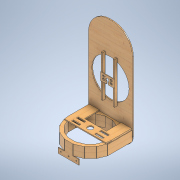
# Autodesk Inventor part: Aufbau
Saved by Autodesk Inventor 2020.3 (Build 243373010, 373A)
## iProperties
Created: 2020-02-10
Part Number: Aufbau
Material: Generisch
Document SubType Name: Modeling
Designer: Stefan
Density: 1 g/cm^3
Appearance: Vorgabe
Mass: 38281.1 g
Surface Area: 55122.2 cm^2
Volume: 38281.1 cm^3
Author: Stefan
Autodesk Inventor part; units mm, degrees
ref_plane "YZ Plane" through (0, 0, 0) normal (1, 0, 0) x (0, 1, 0)
ref_plane "XZ Plane" through (0, 0, 0) normal (0, 1, 0) x (-1, 0, 0)
ref_plane "XY Plane" through (0, 0, 0) normal (0, 0, 1) x (1, 0, 0)
sketch "Skizze1" plane through (0, 0, 0) normal (0, 0, 1) x (-1, 0, 0)
  line L0 (225, 975) -> (-225, 975)
  line L1 (-425, 775) -> (-425, -575)
  line L2 (-25, -975) -> (25, -975)
  line L3 (425, -575) -> (425, 775)
  arc A0 (425, 775) -> (225, 975) centre (225, 775) ccw
  arc A1 (-225, 975) -> (-425, 775) centre (-225, 775) ccw
  arc A2 (-425, -575) -> (-25, -975) centre (-25, -575) ccw
  arc A3 (25, -975) -> (425, -575) centre (25, -575) ccw
  circle A4 centre (0, 0) radius 360
  point P0 (425, 975)
  point P1 (-425, 975)
  point P2 (425, -975)
  dimension "d0" = 850
  dimension "d1" = 1950
  dimension "d2" = 975
  dimension "d3" = 425
  dimension "d4" = 200
  dimension "d5" = 200
  dimension "d6" = 400
  dimension "d7" = 400
  dimension "d8" = 720
  constraints: 8 end point, 8 point on circle, 8 tangent, 6 point on line, 5 centre point, 2 parallel, 1 coincident, 1 horizontal, 1 perpendicular
  measures "d0" distance of point (425, 975) point (-425, 975)
  measures "d1" distance of point (425, -975) point (425, 975)
  measures "d2" distance from line of L2 point (0, 0)
  measures "d3" distance from line of L3 point (0, 0)
  measures "d4" radius of A0
  measures "d5" radius of A1
  measures "d6" radius of A2
  measures "d7" radius of A3
  measures "d8" diameter of A4
extrude "Extrusion1" add sketch "Skizze1" along normal blind 18
sketch "Skizze36" plane through (0, 0, 18) normal (0, 0, 1) x (1, 0, 0)
  line L0 (-130, -400) -> (-100, -400)
  line L1 (-100, -400) -> (-100, 400)
  line L2 (-100, 400) -> (-130, 400)
  line L3 (-130, 400) -> (-130, -400)
  line L4 (100, -400) -> (130, -400)
  line L5 (130, -400) -> (130, 400)
  line L6 (130, 400) -> (100, 400)
  line L7 (100, 400) -> (100, -400)
  point P0 (0, 0)
  dimension "d196" = 30
  dimension "d197" = 30
  dimension "d198" = 100
  dimension "d199" = 100
  dimension "d200" = 800
  dimension "d201" = 400
  dimension "d202" = 0
  dimension "d203" = 0
  constraints: 16 end point, 4 parallel, 2 horizontal, 2 perpendicular
  measures "d196" distance of L1.end L2.end
  measures "d197" distance of L5.end L6.end
  measures "d198" distance from line of point (0, 0) L1
  measures "d199" distance from line of point (0, 0) L7
  measures "d200" distance of L6.end L4.start
  measures "d201" distance from line of point (0, 0) L4
  measures "d202" distance between parallel lines of L4 L0
  measures "d203" distance between parallel lines of L6 L2
extrude "Extrusion30" add sketch "Skizze36" along normal blind 50
sketch "Skizze38" plane through (0, 0, 68) normal (0, 0, 1) x (1, 0, 0)
  line L0 (15, -75) -> (130, -75)
  line L1 (130, -75) -> (130, 75)
  line L2 (130, 75) -> (-130, 75)
  line L3 (-130, 75) -> (-130, -75)
  line L4 (-130, -75) -> (-15, -75)
  circle A0 centre (35.0018, 35.0018) radius 3.1
  circle A1 centre (35.0018, -35.0018) radius 3.1
  circle A2 centre (-35.0018, -35.0018) radius 3.1
  circle A3 centre (-35.0018, 35.0018) radius 3.1
  arc A4 (15, -25.9808) -> (-15, -25.9808) centre (0, 0) ccw
  line L5 (15, -25.9808) -> (15, -75)
  line L6 (-15, -25.9808) -> (-15, -75)
  line L7 (-95, -16.5909) -> (-95, -38.4091)
  line L8 (-87.3733, -10) -> (-74.75, -20.9091)
  line L9 (-62.1267, -45) -> (-74.75, -34.0909)
  line L10 (-95, -38.4091) -> (-82.3767, -27.5)
  line L11 (-87.3733, -45) -> (-74.75, -34.0909)
  line L12 (-74.75, -20.9091) -> (-62.1267, -10)
  line L13 (-82.3767, -27.5) -> (-95, -16.5909)
  line L14 (-67.1233, -27.5) -> (-54.5, -16.5909)
  line L15 (-67.1233, -27.5) -> (-54.5, -38.4091)
  line L16 (-54.5, -38.4091) -> (-54.5, -16.5909)
  line L17 (-87.3733, -45) -> (-62.1267, -45)
  line L18 (-62.1267, -10) -> (-87.3733, -10)
  line L19 (-95, 16.5909) -> (-95, 38.4091)
  line L20 (-87.3733, 45) -> (-62.1267, 45)
  line L21 (-54.5, 38.4091) -> (-54.5, 16.5909)
  line L22 (-62.1267, 10) -> (-87.3733, 10)
  line L23 (-87.3733, 10) -> (-74.75, 20.9091)
  line L24 (-67.1233, 27.5) -> (-54.5, 38.4091)
  line L25 (-62.1267, 45) -> (-74.75, 34.0909)
  line L26 (-82.3767, 27.5) -> (-95, 16.5909)
  line L27 (-95, 38.4091) -> (-82.3767, 27.5)
  line L28 (-74.75, 20.9091) -> (-62.1267, 10)
  line L29 (-87.3733, 45) -> (-74.75, 34.0909)
  line L30 (-67.1233, 27.5) -> (-54.5, 16.5909)
  line L31 (95, -16.5909) -> (95, -38.4091)
  line L32 (87.3733, -45) -> (62.1267, -45)
  line L33 (54.5, -38.4091) -> (54.5, -16.5909)
  line L34 (62.1267, -10) -> (87.3733, -10)
  line L35 (87.3733, -10) -> (74.75, -20.9091)
  line L36 (67.1233, -27.5) -> (54.5, -38.4091)
  line L37 (62.1267, -45) -> (74.75, -34.0909)
  line L38 (82.3767, -27.5) -> (95, -16.5909)
  line L39 (95, -38.4091) -> (82.3767, -27.5)
  line L40 (74.75, -20.9091) -> (62.1267, -10)
  line L41 (87.3733, -45) -> (74.75, -34.0909)
  line L42 (67.1233, -27.5) -> (54.5, -16.5909)
  line L43 (95, 16.5909) -> (95, 38.4091)
  line L44 (87.3733, 45) -> (62.1267, 45)
  line L45 (54.5, 38.4091) -> (54.5, 16.5909)
  line L46 (62.1267, 10) -> (87.3733, 10)
  line L47 (87.3733, 10) -> (74.75, 20.9091)
  line L48 (67.1233, 27.5) -> (54.5, 38.4091)
  line L49 (62.1267, 45) -> (74.75, 34.0909)
  line L50 (82.3767, 27.5) -> (95, 16.5909)
  line L51 (95, 38.4091) -> (82.3767, 27.5)
  line L52 (74.75, 20.9091) -> (62.1267, 10)
  line L53 (87.3733, 45) -> (74.75, 34.0909)
  line L54 (67.1233, 27.5) -> (54.5, 16.5909)
  point P0 (0, 0)
  point P1 (15, -25.9808)
  point P2 (130, 75)
  point P3 (-130, -75)
  point P4 (-15, -25.9808)
  constraints: 110 end point, 5 centre point, 2 point on circle
extrude "Extrusion32" add sketch "Skizze38" along normal blind 10
sketch "Skizze48" plane through (0, 0, 18) normal (0, 0, 1) x (1, 0, 0)
  line L0 (-410, -855) -> (410, -855)
  line L1 (410, -855) -> (410, -845)
  line L2 (410, -845) -> (-410, -845)
  line L3 (-410, -845) -> (-410, -855)
  line L4 (-425, 575) -> (-425, -775) projected
  line L5 (425, -775) -> (425, 575) projected
  line L6 (-225, -975) -> (225, -975) projected
  line L7 (-410, -665) -> (410, -665)
  line L8 (410, -665) -> (410, -655)
  line L9 (410, -655) -> (-410, -655)
  line L10 (-410, -655) -> (-410, -665)
  point P0 (0, 0)
  point P1 (425, -641)
  point P2 (-425, -641)
  point P3 (-425, -648)
  point P4 (425, -648)
  dimension "d300" = 10
  dimension "d302" = 15
  dimension "d304" = 120
  dimension "d308" = 10
  dimension "d309" = 820
  dimension "d310" = 180
  dimension "d314" = 820
  dimension "d315" = 15
  dimension "d316" = 0
  dimension "d317" = 0
  constraints: 16 end point, 4 parallel, 2 horizontal, 2 perpendicular
  measures "d300" distance of L2.end L0.start
  measures "d302" distance between parallel lines of L5 L1
  measures "d304" distance between parallel lines of L6 L0
  measures "d308" distance between parallel lines of L9 L7
  measures "d309" distance of L7.start L7.end
  measures "d310" distance between parallel lines of L2 L7
  measures "d314" distance of L0.start L0.end
  measures "d315" distance between parallel lines of L4 L3
  measures "d316" distance between parallel lines of L3 L10
  measures "d317" distance between parallel lines of L1 L8
extrude "Extrusion40" add sketch "Skizze48" along normal blind 800
sketch "Skizze50" plane through (-410, -655, 18) normal (0, 1, 0) x (1, 0, 0)
  line L0 (820, 0) -> (0, 0) projected
  line L1 (820, 0) -> (620, 0)
  line L2 (620, 0) -> (620, -290)
  line L3 (620, -290) -> (820, -290)
  line L4 (820, -290) -> (820, 0)
  line L5 (0, 0) -> (200, 0)
  line L6 (200, 0) -> (200, -290)
  line L7 (200, -290) -> (0, -290)
  line L8 (0, -290) -> (0, 0)
  line L9 (0, 0) -> (0, -800) projected
  line L10 (820, -290) -> (0, -290)
  line L11 (0, -390) -> (0, -290)
  line L12 (820, 0) -> (820, -800) projected
  line L13 (820, -290) -> (820, -390)
  arc A0 (0, -390) -> (820, -390) centre (410, -390) ccw
  arc A1 (807.6179, -490) -> (820, -390) centre (410, -390) ccw
  arc A2 (0, -390) -> (12.3821, -490) centre (410, -390) ccw
  line L14 (12.3821, -490) -> (807.6179, -490)
  circle A3 centre (410, -390) radius 50
  line L15 (710, -455) -> (560, -455)
  line L16 (560, -455) -> (560, -420)
  line L17 (560, -420) -> (710, -420)
  line L18 (710, -420) -> (710, -455)
  line L19 (710, -325) -> (560, -325)
  line L20 (560, -325) -> (560, -360)
  line L21 (560, -360) -> (710, -360)
  line L22 (710, -360) -> (710, -325)
  line L23 (410, -290) -> (410, -490) construction
  line L24 (110, -455) -> (260, -455)
  line L25 (260, -455) -> (260, -420)
  line L26 (260, -420) -> (110, -420)
  line L27 (110, -420) -> (110, -455)
  line L28 (110, -325) -> (260, -325)
  line L29 (260, -325) -> (260, -360)
  line L30 (260, -360) -> (110, -360)
  line L31 (110, -360) -> (110, -325)
  point P0 (410, 18)
  point P1 (200, 0)
  point P2 (200, -290)
  dimension "d323" = 200
  dimension "d324" = 290
  dimension "d325" = 200
  dimension "d326" = 290
  dimension "d331" = 100
  dimension "d332" = 100
  dimension "d333" = 100
  dimension "d334" = 150
  dimension "d335" = 35
  dimension "d336" = 35
  dimension "d337" = 150
  dimension "d338" = 35
  dimension "d339" = 35
  dimension "d340" = 150
  dimension "d341" = 0
  dimension "d342" = 60
  constraints: 58 end point, 8 parallel, 8 point on circle, 8 symmetric about line, 4 centre point, 4 horizontal, 4 perpendicular, 2 coincident, 2 midpoint, 1 collinear, 1 concentric
  measures "d323" distance of L3.end L2.end
  measures "d324" distance of L3.end L0.start
  measures "d325" distance of L6.end L7.end
  measures "d326" distance of L5.end L6.end
  measures "d331" vertical distance of L13.end L14.end
  measures "d332" vertical distance of L11.start L14.start
  measures "d333" diameter of A3
  measures "d334" distance of L16.end L17.end
  measures "d335" distance of L15.end L16.end
  measures "d336" distance from line of L14 L15.end
  measures "d337" distance of L21.end L20.end
  measures "d338" distance of L20.end L19.end
  measures "d339" distance from line of L10 L19.start
  measures "d340" distance from line of A1.centre L16
  measures "d341" distance between parallel lines of L22 L18
  measures "d342" distance between parallel lines of L21 L17
extrude "Extrusion42" add sketch "Skizze50" along normal blind 18 contours L4 L3 L2 L0 | L6 L7 L8 L0
extrude "Extrusion43" add sketch "Skizze50" along normal blind 18 contours L12 A0 L14 L9 L7 L10 L3
sketch "Skizze51" plane through (-408.303, -855, 18) normal (0, -1, 0) x (1, 0, 0)
  line L0 (617.8912, 703.6709) -> (721.9739, 599.5882)
  line L1 (721.9739, 599.5882) -> (778.303, 463.5976)
  line L2 (778.303, 463.5976) -> (778.303, 316.4024)
  line L3 (778.303, 316.4024) -> (721.9739, 180.4118)
  line L4 (721.9739, 180.4118) -> (617.8912, 76.3291)
  line L5 (617.8912, 76.3291) -> (481.9006, 20)
  line L6 (481.9006, 20) -> (334.7055, 20)
  line L7 (334.7055, 20) -> (198.7149, 76.3291)
  line L8 (198.7149, 76.3291) -> (94.6322, 180.4118)
  line L9 (94.6322, 180.4118) -> (38.303, 316.4024)
  line L10 (38.303, 316.4024) -> (38.303, 463.5976)
  line L11 (38.303, 463.5976) -> (94.6322, 599.5882)
  line L12 (94.6322, 599.5882) -> (198.7149, 703.6709)
  line L13 (198.7149, 703.6709) -> (334.7055, 760)
  line L14 (334.7055, 760) -> (481.9006, 760)
  line L15 (481.9006, 760) -> (617.8912, 703.6709)
  line L16 (816.6061, 0) -> (0, 0) projected
  line L17 (818.303, 0) -> (818.303, 800) projected
  line L18 (489.8571, 800) -> (640.5494, 737.5812)
  line L19 (640.5494, 737.5812) -> (755.8842, 622.2463)
  line L20 (755.8842, 622.2463) -> (818.303, 471.5541)
  line L21 (-1.697, 471.5541) -> (60.7218, 622.2463)
  line L22 (60.7218, 622.2463) -> (176.0567, 737.5812)
  line L23 (176.0567, 737.5812) -> (326.749, 800)
  line L24 (-1.697, 390) -> (-1.697, 800) projected
  line L25 (-1.697, 471.5541) -> (-1.697, 800)
  line L26 (-1.697, 800) -> (326.749, 800)
  line L27 (489.8571, 800) -> (818.303, 800)
  line L28 (818.303, 471.5541) -> (818.303, 800)
  point P0 (408.303, -18)
  point P1 (408.303, 390)
  point P2 (408.303, 390)
  point P3 (408.303, 800)
  point P4 (818.303, 471.5541)
  dimension "d347" = 390
  dimension "d348" = 410
  dimension "d349" = 0
  dimension "d350" = 370
  constraints: 52 end point, 1 coincident, 1 vertical, 45 other
  measures "d347" distance from line of L16 point (408.303, 390)
  measures "d348" distance from line of L17 point (408.303, 390)
  measures "d349" vertical distance of L13.end L14.end
  measures "d350" distance from line of L10 point (408.303, 390)
extrude "Extrusion44" cut sketch "Skizze51" against normal up to surface (200 mm away)
sketch "Skizze52" plane through (-73.5976, -855, 38) normal (0, 0, 1) x (1, 0, 0)
  line L0 (0, 200) -> (147.1952, 200) projected
  line L1 (147.1952, 0) -> (147.1952, 10) projected
  line L2 (0, 200) -> (147.1952, 200)
  line L3 (147.1952, 200) -> (147.1952, 0)
  line L4 (147.1952, 0) -> (0, 0)
  line L5 (0, 0) -> (0, 200)
  point P0 (73.5976, 855)
  dimension "d403" = 147.1952
  constraints: 8 end point, 2 parallel, 1 horizontal, 1 perpendicular
  measures "d403" distance of L1.start L4.end
extrude "Extrusion45" add sketch "Skizze52" along normal blind 10
pattern_circular "Runde Anordnung1" count 16 over 360 about axis through (0, -655, 408) along (0, 1, 0) of "Extrusion45"
sketch "Skizze53" plane through (-347.5812, -665, 640.2463) normal (-0.9238795, 0, 0.3826834) x (0.3826834, 0, 0.9238795)
  line L0 (-163.1081, 10) -> (0, 10) projected
  line L1 (150.6923, -190) -> (0, -190) projected
  line L2 (-163.1081, 10) -> (0, 10)
  line L3 (0, 10) -> (0, -190)
  line L4 (0, -190) -> (-163.1081, -190)
  line L5 (-163.1081, -190) -> (-163.1081, 10)
  point P0 (-458.4969, 665)
  point P1 (0, 10)
  constraints: 8 end point, 2 parallel, 1 horizontal, 1 perpendicular
extrude "Extrusion46" add sketch "Skizze53" along normal blind 10
pattern_circular "Runde Anordnung2" count 7 over 135 about axis through (0, -655, 408) along (0, 1, 0) of "Extrusion46"
sketch "Skizze57" plane through (-410, -855, 489.5541) normal (-1, 0, 0) x (0, 0, 1)
  line L0 (0, 0) -> (3.8268, 0) projected
  line L1 (0, 0) -> (-471.5541, 0)
  line L2 (-471.5541, 0) -> (-471.5541, 200)
  line L3 (-471.5541, 200) -> (0, 200)
  line L4 (0, 200) -> (0, 0)
  line L5 (-471.5541, 190) -> (-471.5541, 218) projected
  line L6 (-471.5541, 190) -> (0, 190) projected
  point P0 (-489.5541, 855)
  point P1 (-471.5541, 190)
  dimension "d369" = 0
  dimension "d370" = 10
  constraints: 8 end point, 2 parallel, 1 horizontal, 1 perpendicular
  measures "d369" distance between parallel lines of L5 L2
  measures "d370" distance between parallel lines of L6 L3
extrude "Extrusion48" add sketch "Skizze57" along normal blind 10 contours L1 L2 L6 L4
mirror "Spiegeln1" about plane through (0, 0, 0) normal (1, 0, 0) of "Extrusion48"
sketch "Skizze59" plane through (-81.5541, -855, 828) normal (0, 0, 1) x (1, 0, 0)
  line L0 (-118.4459, 0) -> (281.5541, 0)
  line L1 (281.5541, 0) -> (281.5541, -100)
  line L2 (281.5541, -100) -> (-118.4459, -100)
  line L3 (-118.4459, -100) -> (-118.4459, 0)
  line L4 (0, 0) -> (163.1081, 0) projected
  arc A0 (96.5541, 829.0192) -> (66.5541, 829.0192) centre (81.5541, 855) ccw projected
  point P0 (81.5541, 855)
  dimension "d374" = 100
  dimension "d375" = 0
  dimension "d376" = 400
  dimension "d377" = 200
  constraints: 8 end point, 2 parallel, 1 horizontal, 1 perpendicular
  measures "d374" distance of L0.end L1.end
  measures "d375" distance between parallel lines of L0 L4
  measures "d376" distance of L0.start L0.end
  measures "d377" distance from line of A0.centre L1
extrude "Extrusion49" add sketch "Skizze59" against normal blind 10
sketch "Skizze61" plane through (-73.5976, -855, 48) normal (0, 0, 1) x (1, 0, 0)
  line L0 (-126.4024, 0) -> (273.5976, 0)
  line L1 (273.5976, 0) -> (273.5976, -100)
  line L2 (273.5976, -100) -> (-126.4024, -100)
  line L3 (-126.4024, -100) -> (-126.4024, 0)
  line L4 (0, 0) -> (147.1952, 0) projected
  line L5 (273.5976, -100) -> (273.5976, 0) projected
  point P0 (73.5976, 855)
  point P1 (1.9891, 0)
  point P2 (145.206, 0)
  dimension "d391" = 400
  dimension "d392" = 100
  dimension "d393" = 0
  dimension "d394" = 0
  constraints: 8 end point, 2 parallel, 1 horizontal, 1 perpendicular
  measures "d391" distance of L1.end L2.end
  measures "d392" distance of L0.end L1.end
  measures "d393" distance between parallel lines of L4 L0
  measures "d394" distance between parallel lines of L5 L1
extrude "Extrusion51" add sketch "Skizze61" against normal blind 10
sketch "Skizze60" plane through (-81.5541, -655, 828) normal (0, 0, 1) x (1, 0, 0)
  circle A0 centre (81.5541, -250) radius 10
  circle A1 centre (231.5541, -250) radius 10
  circle A2 centre (-68.4459, -250) radius 10
  line L0 (-118.4459, -300) -> (281.5541, -300) projected
  line L1 (-118.4459, -200) -> (-118.4459, -300) projected
  line L2 (281.5541, -300) -> (281.5541, -200) projected
  point P0 (81.5541, 655)
  dimension "d380" = 20
  dimension "d381" = 20
  dimension "d382" = 20
  dimension "d383" = 50
  dimension "d384" = 50
  dimension "d385" = 50
  dimension "d386" = 200
  dimension "d387" = 50
  dimension "d388" = 50
  constraints: 3 centre point
  measures "d380" diameter of A0
  measures "d381" diameter of A1
  measures "d382" diameter of A2
  measures "d383" distance from line of L0 A2.centre
  measures "d384" distance from line of L0 A0.centre
  measures "d385" distance from line of L0 A1.centre
  measures "d386" distance from line of L1 A0.centre
  measures "d387" distance from line of A1.centre L2
  measures "d388" distance from line of L1 A2.centre
extrude "Extrusion50" cut sketch "Skizze60" against normal up to surface (790 mm away)
sketch "Wimkel-16eck" plane through (-71.6085, -655, 768) normal (0, 1, 0) x (1, 0, 0)
  line L0 (143.2169, 0) -> (275.5321, 54.8067) projected
  line L1 (143.2169, 0) -> (0.0166, 0)
  line L2 (0.0166, 0) -> (-75.5064, 31.2827)
  line L3 (0.0166, 0) -> (-3.9649, -20.0167)
  line L4 (0.0166, 0) -> (20.4255, 0) construction
  line L5 (307.6816, 3.18) -> (156.9894, -59.2388) projected
  line L6 (307.6816, 3.18) -> (247.8882, 92.6672)
  line L7 (310.9259, 5.3477) -> (426.2607, 120.6826) projected
  line L8 (310.9259, 5.3477) -> (426.2607, 120.6826)
  line L9 (241.9996, 104.9916) -> (333.5056, -31.9568)
  line L10 (376.8017, 156.0764) -> (419.8483, 260) projected
  line L11 (376.8017, 156.0764) -> (509.4931, 67.4148)
  line L12 (295.4524, -10.1257) -> (446.6083, 141.0302)
  line L13 (309.5193, 3.9412) -> (427.6673, 122.0891)
  point P0 (71.6085, 768)
  dimension "d397" = 157.5
  dimension "d399" = 101.25
  dimension "d400" = 101.25
  dimension "d401" = 78.75
  dimension "d402" = 78.75
  dimension "d404" = 0
  dimension "d405" = 0
  dimension "d406" = 78.75
  dimension "d407" = 180
  dimension "d408" = 167.0864
  constraints: 20 end point, 4 point on line, 2 horizontal, 1 collinear, 1 equal length
  measures "d397" angle of L1 L2
  measures "d399" angle of L3 L4
  measures "d400" angle of L2 L3
  measures "d401" angle of L5 L6
  measures "d402" angle of L6 L7
  measures "d404" angle of L9 L6
  measures "d405" distance from line of L0.end L9
  measures "d406" angle of L11 L7
  measures "d407" angle of L7 L12
  measures "d408" distance of L13.start L13.end
sketch "Skizze63" plane through (-408.303, -855, 18) normal (0, -1, 0) x (1, 0, 0)
  point P0 (408.303, -18)
sketch "Skizze66" plane through (-81.5541, -655, 828) normal (0, 0, 1) x (1, 0, 0)
  circle A0 centre (81.5541, -250) radius 10 projected
  circle A1 centre (81.5541, -250) radius 94
  point P0 (81.5541, 655)
  dimension "d414" = 188
  constraints: 1 centre point, 1 coincident
  measures "d414" diameter of A1
equation "\"dicke\" = 4"
